Autodesk Fusion 360 part; units mm, degrees
(part 2 of 6)
sketch "mv_universal" plane through (-8.3287, 0, 77.2483) normal (0, 1, 0) x (1, 0, 0)
  line L0 (34.3787, 70.2483) -> (34.3787, 84.2483)
  line L1 (53.4287, 84.2483) -> (39.4287, 84.2483)
  line L2 (15.3287, 70.2483) -> (15.3287, 84.2483)
  line L3 (1.3287, 70.2483) -> (15.3287, 70.2483)
  line L4 (39.4287, 70.2483) -> (53.4287, 70.2483)
  line L5 (15.3287, 84.2483) -> (1.3287, 84.2483)
  line L6 (20.3787, 70.2483) -> (34.3787, 70.2483)
  line L7 (34.3787, 84.2483) -> (20.3787, 84.2483)
  line L8 (20.3787, 84.2483) -> (20.3787, 70.2483)
  line L9 (1.3287, 84.2483) -> (1.3287, 70.2483)
  line L10 (153.7287, 70.2483) -> (167.7287, 70.2483)
  line L11 (153.7287, 84.2483) -> (153.7287, 70.2483)
  line L12 (186.7787, 70.2483) -> (186.7787, 84.2483)
  line L13 (172.7787, 84.2483) -> (172.7787, 70.2483)
  line L14 (191.8287, 70.2483) -> (205.8287, 70.2483)
  line L15 (205.8287, 84.2483) -> (191.8287, 84.2483)
  line L16 (72.4787, 70.2483) -> (72.4787, 84.2483)
  line L17 (58.4787, 84.2483) -> (58.4787, 70.2483)
  line L18 (77.5287, 84.2483) -> (77.5287, 70.2483)
  line L19 (110.5787, 70.2483) -> (110.5787, 84.2483)
  line L20 (167.7287, 84.2483) -> (153.7287, 84.2483)
  line L21 (53.4287, 70.2483) -> (53.4287, 84.2483)
  line L22 (167.7287, 70.2483) -> (167.7287, 84.2483)
  line L23 (129.6287, 70.2483) -> (129.6287, 84.2483)
  line L24 (172.7787, 70.2483) -> (186.7787, 70.2483)
  line L25 (186.7787, 84.2483) -> (172.7787, 84.2483)
  line L26 (134.6787, 84.2483) -> (134.6787, 70.2483)
  line L27 (148.6787, 84.2483) -> (134.6787, 84.2483)
  line L28 (58.4787, 70.2483) -> (72.4787, 70.2483)
  line L29 (115.6287, 84.2483) -> (115.6287, 70.2483)
  line L30 (148.6787, 70.2483) -> (148.6787, 84.2483)
  line L31 (39.4287, 84.2483) -> (39.4287, 70.2483)
  line L32 (191.8287, 84.2483) -> (191.8287, 70.2483)
  line L33 (218.0224, 70.2483) -> (232.0224, 70.2483)
  line L34 (3.7099, 51.1983) -> (17.7099, 51.1983)
  line L35 (218.0224, 84.2483) -> (218.0224, 70.2483)
  line L36 (17.7099, 51.1983) -> (17.7099, 65.1983)
  line L37 (96.5787, 84.2483) -> (96.5787, 70.2483)
  line L38 (91.5287, 84.2483) -> (77.5287, 84.2483)
  line L39 (72.4787, 84.2483) -> (58.4787, 84.2483)
  line L40 (115.6287, 70.2483) -> (129.6287, 70.2483)
  line L41 (232.0224, 84.2483) -> (218.0224, 84.2483)
  line L42 (17.7099, 65.1983) -> (3.7099, 65.1983)
  line L43 (96.5787, 70.2483) -> (110.5787, 70.2483)
  line L44 (232.0224, 70.2483) -> (232.0224, 84.2483)
  line L45 (3.7099, 65.1983) -> (3.7099, 51.1983)
  line L46 (134.6787, 70.2483) -> (148.6787, 70.2483)
  line L47 (91.5287, 70.2483) -> (91.5287, 84.2483)
  line L48 (77.5287, 70.2483) -> (91.5287, 70.2483)
  line L49 (129.6287, 84.2483) -> (115.6287, 84.2483)
  line L50 (110.5787, 84.2483) -> (96.5787, 84.2483)
  line L51 (205.8287, 70.2483) -> (205.8287, 84.2483)
  line L52 (158.4912, 51.1983) -> (172.4912, 51.1983)
  line L53 (39.1412, 65.1983) -> (25.1412, 65.1983)
  line L54 (58.1912, 51.1983) -> (58.1912, 65.1983)
  line L55 (82.2912, 51.1983) -> (96.2912, 51.1983)
  line L56 (101.3412, 51.1983) -> (115.3412, 51.1983)
  line L57 (39.1412, 51.1983) -> (39.1412, 65.1983)
  line L58 (44.1912, 65.1983) -> (44.1912, 51.1983)
  line L59 (63.2412, 51.1983) -> (77.2412, 51.1983)
  line L60 (25.1412, 51.1983) -> (39.1412, 51.1983)
  line L61 (77.2412, 65.1983) -> (63.2412, 65.1983)
  line L62 (63.2412, 65.1983) -> (63.2412, 51.1983)
  line L63 (77.2412, 51.1983) -> (77.2412, 65.1983)
  line L64 (82.2912, 65.1983) -> (82.2912, 51.1983)
  line L65 (134.3912, 65.1983) -> (120.3912, 65.1983)
  line L66 (139.4412, 51.1983) -> (153.4412, 51.1983)
  line L67 (153.4412, 65.1983) -> (139.4412, 65.1983)
  line L68 (153.4412, 51.1983) -> (153.4412, 65.1983)
  line L69 (139.4412, 65.1983) -> (139.4412, 51.1983)
  line L70 (172.4912, 65.1983) -> (158.4912, 65.1983)
  line L71 (134.3912, 51.1983) -> (134.3912, 65.1983)
  line L72 (58.1912, 65.1983) -> (44.1912, 65.1983)
  line L73 (101.3412, 65.1983) -> (101.3412, 51.1983)
  line L74 (115.3412, 51.1983) -> (115.3412, 65.1983)
  line L75 (44.1912, 51.1983) -> (58.1912, 51.1983)
  line L76 (96.2912, 65.1983) -> (82.2912, 65.1983)
  line L77 (115.3412, 65.1983) -> (101.3412, 65.1983)
  line L78 (25.1412, 65.1983) -> (25.1412, 51.1983)
  line L79 (120.3912, 65.1983) -> (120.3912, 51.1983)
  line L80 (34.3787, 27.0983) -> (29.9037, 27.0983)
  line L81 (148.9662, 32.1483) -> (162.9662, 32.1483)
  line L82 (220.4037, 51.1983) -> (234.4037, 51.1983)
  line L83 (220.4037, 65.1983) -> (220.4037, 51.1983)
  line L84 (191.5412, 65.1983) -> (177.5412, 65.1983)
  line L85 (172.4912, 51.1983) -> (172.4912, 65.1983)
  line L86 (234.4037, 51.1983) -> (234.4037, 65.1983)
  line L87 (22.4724, 46.1483) -> (8.4724, 46.1483)
  line L88 (177.5412, 51.1983) -> (191.5412, 51.1983)
  line L89 (196.5912, 51.1983) -> (210.5912, 51.1983)
  line L90 (8.4724, 32.1483) -> (22.4724, 32.1483)
  line L91 (96.2912, 51.1983) -> (96.2912, 65.1983)
  line L92 (158.4912, 65.1983) -> (158.4912, 51.1983)
  line L93 (210.5912, 51.1983) -> (210.5912, 65.1983)
  line L94 (196.5912, 65.1983) -> (196.5912, 51.1983)
  line L95 (22.4724, 32.1483) -> (22.4724, 46.1483)
  line L96 (48.6662, 46.1483) -> (34.6662, 46.1483)
  line L97 (239.1662, 46.1483) -> (225.1662, 46.1483)
  line L98 (29.9037, 13.0983) -> (34.3787, 13.0983)
  line L99 (177.5412, 65.1983) -> (177.5412, 51.1983)
  line L100 (234.4037, 65.1983) -> (220.4037, 65.1983)
  line L101 (225.1662, 32.1483) -> (239.1662, 32.1483)
  line L102 (29.9037, 27.0983) -> (20.3787, 27.0983)
  line L103 (20.3787, 27.0983) -> (20.3787, 13.0983)
  line L104 (182.0162, 46.1483) -> (168.0162, 46.1483)
  line L105 (210.5912, 65.1983) -> (196.5912, 65.1983)
  line L106 (34.3787, 13.0983) -> (39.4287, 13.0983)
  line L107 (15.3287, 13.0983) -> (17.7099, 13.0983)
  line L108 (17.7099, 13.0983) -> (17.7099, 27.0983)
  line L109 (120.3912, 51.1983) -> (134.3912, 51.1983)
  line L110 (191.5412, 51.1983) -> (191.5412, 65.1983)
  line L111 (143.9162, 46.1483) -> (129.9162, 46.1483)
  line L112 (220.1162, 32.1483) -> (220.1162, 46.1483)
  line L113 (34.6662, 32.1483) -> (48.6662, 32.1483)
  line L114 (225.1662, 46.1483) -> (225.1662, 32.1483)
  line L115 (53.7162, 46.1483) -> (53.7162, 32.1483)
  line L116 (67.7162, 46.1483) -> (53.7162, 46.1483)
  line L117 (43.9037, 27.0983) -> (39.4287, 27.0983)
  line L118 (91.8162, 46.1483) -> (91.8162, 32.1483)
  line L119 (3.7099, 13.0983) -> (15.3287, 13.0983)
  line L120 (129.9162, 46.1483) -> (129.9162, 32.1483)
  line L121 (162.9662, 32.1483) -> (162.9662, 46.1483)
  line L122 (15.3287, 27.0983) -> (3.7099, 27.0983)
  line L123 (168.0162, 32.1483) -> (182.0162, 32.1483)
  line L124 (187.0662, 46.1483) -> (187.0662, 32.1483)
  line L125 (206.1162, 46.1483) -> (206.1162, 32.1483)
  line L126 (86.7662, 46.1483) -> (72.7662, 46.1483)
  line L127 (201.0662, 46.1483) -> (187.0662, 46.1483)
  line L128 (17.7099, 27.0983) -> (15.3287, 27.0983)
  line L129 (3.7099, 27.0983) -> (1.3287, 27.0983)
  line L130 (8.4724, 46.1483) -> (8.4724, 32.1483)
  line L131 (67.7162, 32.1483) -> (67.7162, 46.1483)
  line L132 (91.8162, 32.1483) -> (105.8162, 32.1483)
  line L133 (129.9162, 32.1483) -> (143.9162, 32.1483)
  line L134 (162.9662, 46.1483) -> (148.9662, 46.1483)
  line L135 (220.1162, 46.1483) -> (206.1162, 46.1483)
  line L136 (239.1662, 32.1483) -> (239.1662, 46.1483)
  line L137 (110.8662, 32.1483) -> (124.8662, 32.1483)
  line L138 (53.4287, 27.0983) -> (43.9037, 27.0983)
  line L139 (201.0662, 32.1483) -> (201.0662, 46.1483)
  line L140 (86.7662, 32.1483) -> (86.7662, 46.1483)
  line L141 (72.7662, 32.1483) -> (86.7662, 32.1483)
  line L142 (53.7162, 32.1483) -> (67.7162, 32.1483)
  line L143 (72.7662, 46.1483) -> (72.7662, 32.1483)
  line L144 (187.0662, 32.1483) -> (201.0662, 32.1483)
  line L145 (1.3287, 27.0983) -> (1.3287, 13.0983)
  line L146 (105.8162, 46.1483) -> (91.8162, 46.1483)
  line L147 (34.6662, 46.1483) -> (34.6662, 32.1483)
  line L148 (43.9037, 13.0983) -> (53.4287, 13.0983)
  line L149 (182.0162, 32.1483) -> (182.0162, 46.1483)
  line L150 (48.6662, 32.1483) -> (48.6662, 46.1483)
  line L151 (1.3287, 13.0983) -> (3.7099, 13.0983)
  line L152 (124.8662, 46.1483) -> (110.8662, 46.1483)
  line L153 (148.9662, 46.1483) -> (148.9662, 32.1483)
  line L154 (168.0162, 46.1483) -> (168.0162, 32.1483)
  line L155 (39.4287, 27.0983) -> (34.3787, 27.0983)
  line L156 (105.8162, 32.1483) -> (105.8162, 46.1483)
  line L157 (124.8662, 32.1483) -> (124.8662, 46.1483)
  line L158 (206.1162, 32.1483) -> (220.1162, 32.1483)
  line L159 (39.4287, 13.0983) -> (43.9037, 13.0983)
  line L160 (143.9162, 32.1483) -> (143.9162, 46.1483)
  line L161 (232.0224, 27.0983) -> (225.1662, 27.0983)
  line L162 (104.8729, 28.0983) -> (104.8729, 13.0983)
  line L163 (111.8729, 28.0983) -> (104.8729, 28.0983)
  line L164 (187.0662, 27.0983) -> (187.0662, 13.0983)
  line L165 (206.1162, 13.0983) -> (218.0224, 13.0983)
  line L166 (220.1162, 27.0983) -> (218.0224, 27.0983)
  line L167 (70.0974, 13.0983) -> (72.4787, 13.0983)
  line L168 (177.2537, 27.0983) -> (174.8724, 27.0983)
  line L169 (53.4287, 13.0983) -> (53.4287, 27.0983)
  line L170 (104.8729, 13.0983) -> (111.8729, 13.0983)
  line L171 (87.9969, 28.0983) -> (80.9969, 28.0983)
  line L172 (110.8662, 46.1483) -> (110.8662, 32.1483)
  line L173 (80.9969, 13.0983) -> (87.9969, 13.0983)
  line L174 (87.9969, 13.0983) -> (87.9969, 28.0983)
  line L175 (143.9162, 27.0983) -> (129.9162, 27.0983)
  line L176 (56.0974, 27.0983) -> (56.0974, 13.0983)
  line L177 (143.9162, 13.0983) -> (143.9162, 27.0983)
  line L178 (218.0224, 13.0983) -> (220.1162, 13.0983)
  line L179 (129.9162, 13.0983) -> (143.9162, 13.0983)
  line L180 (225.1662, 27.0983) -> (220.1162, 27.0983)
  line L181 (20.3787, 13.0983) -> (29.9037, 13.0983)
  line L182 (177.2537, 13.0983) -> (177.2537, 27.0983)
  line L183 (160.8724, 27.0983) -> (160.8724, 13.0983)
  line L184 (152.3542, 28.0983) -> (145.3542, 28.0983)
  line L185 (80.9969, 28.0983) -> (80.9969, 13.0983)
  line L186 (129.9162, 27.0983) -> (129.9162, 13.0983)
  line L187 (103.4349, 27.0983) -> (89.4349, 27.0983)
  line L188 (145.3542, 28.0983) -> (145.3542, 13.0983)
  line L189 (70.0974, 27.0983) -> (58.4787, 27.0983)
  line L190 (163.2537, 13.0983) -> (174.8724, 13.0983)
  line L191 (111.8729, 13.0983) -> (111.8729, 28.0983)
  line L192 (128.4782, 28.0983) -> (121.4782, 28.0983)
  line L193 (201.0662, 27.0983) -> (187.0662, 27.0983)
  line L194 (218.0224, 27.0983) -> (206.1162, 27.0983)
  line L195 (201.0662, 13.0983) -> (201.0662, 27.0983)
  line L196 (103.4349, 13.0983) -> (103.4349, 27.0983)
  line L197 (121.4782, 13.0983) -> (128.4782, 13.0983)
  line L198 (206.1162, 27.0983) -> (206.1162, 13.0983)
  line L199 (58.4787, 13.0983) -> (70.0974, 13.0983)
  line L200 (239.1662, 27.0983) -> (232.0224, 27.0983)
  line L201 (187.0662, 13.0983) -> (201.0662, 13.0983)
  line L202 (145.3542, 13.0983) -> (152.3542, 13.0983)
  line L203 (72.4787, 13.0983) -> (72.4787, 27.0983)
  line L204 (152.3542, 13.0983) -> (152.3542, 28.0983)
  line L205 (174.8724, 13.0983) -> (177.2537, 13.0983)
  line L206 (58.4787, 27.0983) -> (56.0974, 27.0983)
  line L207 (225.1662, 13.0983) -> (232.0224, 13.0983)
  line L208 (56.0974, 13.0983) -> (58.4787, 13.0983)
  line L209 (89.4349, 27.0983) -> (89.4349, 13.0983)
  line L210 (72.4787, 27.0983) -> (70.0974, 27.0983)
  line L211 (232.0224, 13.0983) -> (239.1662, 13.0983)
  line L212 (121.4782, 28.0983) -> (121.4782, 13.0983)
  line L213 (239.1662, 13.0983) -> (239.1662, 27.0983)
  line L214 (89.4349, 13.0983) -> (103.4349, 13.0983)
  line L215 (163.2537, 27.0983) -> (160.8724, 27.0983)
  line L216 (128.4782, 13.0983) -> (128.4782, 28.0983)
  line L217 (174.8724, 27.0983) -> (163.2537, 27.0983)
  line L218 (220.1162, 13.0983) -> (225.1662, 13.0983)
  line L219 (160.8724, 13.0983) -> (163.2537, 13.0983)
  point P0 (8.3287, 77.2483)
sketch "monorail_steam" plane through (-2.7257, 0, 77.6837) normal (0, 1, 0) x (1, 0, 0)
  line L0 (228.8007, 51.6337) -> (228.8007, 65.6337)
  line L1 (43.0632, 32.5837) -> (43.0632, 46.5837)
  line L2 (188.3195, 27.5337) -> (176.7007, 27.5337)
  line L3 (29.0632, 46.5837) -> (29.0632, 32.5837)
  line L4 (138.3132, 32.5837) -> (138.3132, 46.5837)
  line L5 (157.3632, 32.5837) -> (157.3632, 46.5837)
  line L6 (119.2632, 46.5837) -> (105.2632, 46.5837)
  line L7 (209.7507, 27.5337) -> (195.7507, 27.5337)
  line L8 (190.7007, 27.5337) -> (188.3195, 27.5337)
  line L9 (217.182, 27.5337) -> (217.182, 13.5337)
  line L10 (195.7507, 13.5337) -> (209.7507, 13.5337)
  line L11 (190.7007, 13.5337) -> (190.7007, 27.5337)
  line L12 (118.2882, 28.5337) -> (118.2882, 27.5337)
  line L13 (174.3195, 13.5337) -> (176.7007, 13.5337)
  line L14 (231.182, 13.5337) -> (231.182, 27.5337)
  line L15 (217.182, 13.5337) -> (231.182, 13.5337)
  line L16 (174.3195, 27.5337) -> (174.3195, 13.5337)
  line L17 (231.182, 27.5337) -> (217.182, 27.5337)
  line L18 (188.3195, 13.5337) -> (190.7007, 13.5337)
  line L19 (125.2882, 13.5337) -> (125.2882, 28.5337)
  line L20 (195.7507, 27.5337) -> (195.7507, 13.5337)
  line L21 (176.7007, 13.5337) -> (188.3195, 13.5337)
  line L22 (209.7507, 13.5337) -> (209.7507, 27.5337)
  line L23 (176.7007, 27.5337) -> (174.3195, 27.5337)
  line L24 (105.2632, 32.5837) -> (119.2632, 32.5837)
  line L25 (2.8695, 32.5837) -> (16.8695, 32.5837)
  line L26 (162.4132, 32.5837) -> (176.4132, 32.5837)
  line L27 (204.9882, 65.6337) -> (190.9882, 65.6337)
  line L28 (176.4132, 46.5837) -> (162.4132, 46.5837)
  line L29 (62.1132, 46.5837) -> (48.1132, 46.5837)
  line L30 (124.3132, 46.5837) -> (124.3132, 32.5837)
  line L31 (62.1132, 32.5837) -> (62.1132, 46.5837)
  line L32 (195.4632, 46.5837) -> (181.4632, 46.5837)
  line L33 (138.3132, 46.5837) -> (124.3132, 46.5837)
  line L34 (48.1132, 46.5837) -> (48.1132, 32.5837)
  line L35 (105.2632, 46.5837) -> (105.2632, 32.5837)
  line L36 (166.8882, 51.6337) -> (166.8882, 65.6337)
  line L37 (67.1632, 32.5837) -> (81.1632, 32.5837)
  line L38 (171.9382, 51.6337) -> (185.9382, 51.6337)
  line L39 (100.2132, 32.5837) -> (100.2132, 46.5837)
  line L40 (219.5632, 32.5837) -> (233.5632, 32.5837)
  line L41 (176.4132, 32.5837) -> (176.4132, 46.5837)
  line L42 (181.4632, 32.5837) -> (195.4632, 32.5837)
  line L43 (100.2132, 46.5837) -> (86.2132, 46.5837)
  line L44 (200.5132, 32.5837) -> (214.5132, 32.5837)
  line L45 (162.4132, 46.5837) -> (162.4132, 32.5837)
  line L46 (190.9882, 65.6337) -> (190.9882, 51.6337)
  line L47 (29.0632, 32.5837) -> (43.0632, 32.5837)
  line L48 (86.2132, 46.5837) -> (86.2132, 32.5837)
  line L49 (43.0632, 46.5837) -> (29.0632, 46.5837)
  line L50 (185.9382, 51.6337) -> (185.9382, 65.6337)
  line L51 (171.9382, 65.6337) -> (171.9382, 51.6337)
  line L52 (16.8695, 32.5837) -> (16.8695, 46.5837)
  line L53 (124.3132, 32.5837) -> (138.3132, 32.5837)
  line L54 (185.9382, 65.6337) -> (171.9382, 65.6337)
  line L55 (81.1632, 32.5837) -> (81.1632, 46.5837)
  line L56 (228.8007, 65.6337) -> (214.8007, 65.6337)
  line L57 (166.8882, 65.6337) -> (152.8882, 65.6337)
  line L58 (57.6382, 65.6337) -> (57.6382, 51.6337)
  line L59 (133.8382, 65.6337) -> (133.8382, 51.6337)
  line L60 (152.8882, 51.6337) -> (166.8882, 51.6337)
  line L61 (133.8382, 51.6337) -> (147.8382, 51.6337)
  line L62 (90.6882, 65.6337) -> (76.6882, 65.6337)
  line L63 (76.6882, 65.6337) -> (76.6882, 51.6337)
  line L64 (95.7382, 51.6337) -> (109.7382, 51.6337)
  line L65 (109.7382, 65.6337) -> (95.7382, 65.6337)
  line L66 (95.7382, 65.6337) -> (95.7382, 51.6337)
  line L67 (128.7882, 51.6337) -> (128.7882, 65.6337)
  line L68 (147.8382, 51.6337) -> (147.8382, 65.6337)
  line L69 (214.8007, 65.6337) -> (214.8007, 51.6337)
  line L70 (114.7882, 65.6337) -> (114.7882, 51.6337)
  line L71 (109.7382, 51.6337) -> (109.7382, 65.6337)
  line L72 (128.7882, 65.6337) -> (114.7882, 65.6337)
  line L73 (90.6882, 51.6337) -> (90.6882, 65.6337)
  line L74 (114.7882, 51.6337) -> (128.7882, 51.6337)
  line L75 (147.8382, 65.6337) -> (133.8382, 65.6337)
  line L76 (76.6882, 51.6337) -> (90.6882, 51.6337)
  line L77 (143.3632, 46.5837) -> (143.3632, 32.5837)
  line L78 (195.4632, 32.5837) -> (195.4632, 46.5837)
  line L79 (143.3632, 32.5837) -> (157.3632, 32.5837)
  line L80 (181.4632, 46.5837) -> (181.4632, 32.5837)
  line L81 (16.8695, 46.5837) -> (2.8695, 46.5837)
  line L82 (152.8882, 65.6337) -> (152.8882, 51.6337)
  line L83 (214.8007, 51.6337) -> (228.8007, 51.6337)
  line L84 (214.5132, 46.5837) -> (200.5132, 46.5837)
  line L85 (157.3632, 46.5837) -> (143.3632, 46.5837)
  line L86 (67.1632, 46.5837) -> (67.1632, 32.5837)
  line L87 (190.9882, 51.6337) -> (204.9882, 51.6337)
  line L88 (214.5132, 32.5837) -> (214.5132, 46.5837)
  line L89 (86.2132, 32.5837) -> (100.2132, 32.5837)
  line L90 (81.1632, 46.5837) -> (67.1632, 46.5837)
  line L91 (119.2632, 32.5837) -> (119.2632, 46.5837)
  line L92 (200.5132, 46.5837) -> (200.5132, 32.5837)
  line L93 (233.5632, 46.5837) -> (219.5632, 46.5837)
  line L94 (219.5632, 46.5837) -> (219.5632, 32.5837)
  line L95 (204.9882, 51.6337) -> (204.9882, 65.6337)
  line L96 (2.8695, 46.5837) -> (2.8695, 32.5837)
  line L97 (233.5632, 32.5837) -> (233.5632, 46.5837)
  line L98 (48.1132, 32.5837) -> (62.1132, 32.5837)
  line L99 (110.0257, 70.6837) -> (124.0257, 70.6837)
  line L100 (181.1757, 84.6837) -> (167.1757, 84.6837)
  line L101 (85.9257, 84.6837) -> (71.9257, 84.6837)
  line L102 (124.0257, 70.6837) -> (124.0257, 84.6837)
  line L103 (129.0757, 70.6837) -> (143.0757, 70.6837)
  line L104 (162.1257, 70.6837) -> (162.1257, 84.6837)
  line L105 (52.8757, 70.6837) -> (66.8757, 70.6837)
  line L106 (28.7757, 84.6837) -> (14.7757, 84.6837)
  line L107 (162.1257, 84.6837) -> (148.1257, 84.6837)
  line L108 (-4.2743, 70.6837) -> (9.7257, 70.6837)
  line L109 (28.7757, 70.6837) -> (28.7757, 84.6837)
  line L110 (148.1257, 84.6837) -> (148.1257, 70.6837)
  line L111 (167.1757, 84.6837) -> (167.1757, 70.6837)
  line L112 (71.9257, 70.6837) -> (85.9257, 70.6837)
  line L113 (47.8257, 70.6837) -> (47.8257, 84.6837)
  line L114 (85.9257, 70.6837) -> (85.9257, 84.6837)
  line L115 (90.9757, 70.6837) -> (104.9757, 70.6837)
  line L116 (14.7757, 84.6837) -> (14.7757, 70.6837)
  line L117 (71.9257, 84.6837) -> (71.9257, 70.6837)
  line L118 (52.8757, 84.6837) -> (52.8757, 70.6837)
  line L119 (104.9757, 84.6837) -> (90.9757, 84.6837)
  line L120 (110.0257, 84.6837) -> (110.0257, 70.6837)
  line L121 (90.9757, 84.6837) -> (90.9757, 70.6837)
  line L122 (104.9757, 70.6837) -> (104.9757, 84.6837)
  line L123 (47.8257, 84.6837) -> (33.8257, 84.6837)
  line L124 (212.4195, 70.6837) -> (226.4195, 70.6837)
  line L125 (226.4195, 84.6837) -> (212.4195, 84.6837)
  line L126 (226.4195, 70.6837) -> (226.4195, 84.6837)
  line L127 (200.2257, 70.6837) -> (200.2257, 84.6837)
  line L128 (186.2257, 84.6837) -> (186.2257, 70.6837)
  line L129 (-1.893, 51.6337) -> (12.107, 51.6337)
  line L130 (12.107, 51.6337) -> (12.107, 65.6337)
  line L131 (33.5382, 65.6337) -> (19.5382, 65.6337)
  line L132 (19.5382, 65.6337) -> (19.5382, 51.6337)
  line L133 (38.5882, 51.6337) -> (52.5882, 51.6337)
  line L134 (212.4195, 84.6837) -> (212.4195, 70.6837)
  line L135 (-1.893, 65.6337) -> (-1.893, 51.6337)
  line L136 (12.107, 65.6337) -> (-1.893, 65.6337)
  line L137 (19.5382, 51.6337) -> (33.5382, 51.6337)
  line L138 (33.5382, 51.6337) -> (33.5382, 65.6337)
  line L139 (52.5882, 65.6337) -> (38.5882, 65.6337)
  line L140 (38.5882, 65.6337) -> (38.5882, 51.6337)
  line L141 (52.5882, 51.6337) -> (52.5882, 65.6337)
  line L142 (71.6382, 65.6337) -> (57.6382, 65.6337)
  line L143 (57.6382, 51.6337) -> (71.6382, 51.6337)
  line L144 (71.6382, 51.6337) -> (71.6382, 65.6337)
  line L145 (9.7257, 70.6837) -> (9.7257, 84.6837)
  line L146 (33.8257, 84.6837) -> (33.8257, 70.6837)
  line L147 (14.7757, 70.6837) -> (28.7757, 70.6837)
  line L148 (66.8757, 70.6837) -> (66.8757, 84.6837)
  line L149 (61.1445, 13.5337) -> (68.1382, 13.5337)
  line L150 (118.2882, 13.5337) -> (121.6445, 13.5337)
  line L151 (33.5382, 13.5337) -> (33.5382, 27.5337)
  line L152 (76.6882, 13.5337) -> (77.6315, 13.5337)
  line L153 (19.5382, 27.5337) -> (17.157, 27.5337)
  line L154 (168.1445, 13.5337) -> (168.1445, 28.5337)
  line L155 (121.6445, 13.5337) -> (125.2882, 13.5337)
  line L156 (38.5882, 27.5337) -> (38.5882, 13.5337)
  line L157 (106.2382, 28.5337) -> (101.5075, 28.5337)
  line L158 (61.1382, 28.5337) -> (61.1382, 13.5337)
  line L159 (156.3882, 13.5337) -> (161.1445, 13.5337)
  line L160 (133.8382, 27.5337) -> (133.8382, 13.5337)
  line L161 (33.5382, 27.5337) -> (31.157, 27.5337)
  line L162 (61.1445, 28.5337) -> (61.1382, 28.5337)
  line L163 (156.3882, 28.5337) -> (156.3882, 13.5337)
  line L164 (125.2882, 28.5337) -> (118.2882, 28.5337)
  line L165 (161.1445, 28.5337) -> (156.3882, 28.5337)
  line L166 (61.1382, 13.5337) -> (61.1445, 13.5337)
  line L167 (107.6445, 13.5337) -> (118.2882, 13.5337)
  line L168 (147.8382, 27.5337) -> (133.8382, 27.5337)
  line L169 (-4.2743, 27.5337) -> (-4.2743, 13.5337)
  line L170 (94.5075, 28.5337) -> (94.5075, 13.5337)
  line L171 (54.9695, 13.5337) -> (54.9695, 27.5337)
  line L172 (68.1445, 28.5337) -> (68.1382, 28.5337)
  line L173 (77.6315, 28.5337) -> (70.6315, 28.5337)
  line L174 (99.2382, 28.5337) -> (94.5075, 28.5337)
  line L175 (17.157, 27.5337) -> (17.157, 13.5337)
  line L176 (40.9695, 27.5337) -> (38.5882, 27.5337)
  line L177 (40.9695, 13.5337) -> (52.5882, 13.5337)
  line L178 (118.2882, 27.5337) -> (107.6445, 27.5337)
  line L179 (168.1445, 28.5337) -> (163.3882, 28.5337)
  line L180 (31.157, 13.5337) -> (33.5382, 13.5337)
  line L181 (101.5075, 13.5337) -> (106.2382, 13.5337)
  line L182 (107.6445, 27.5337) -> (107.6445, 13.5337)
  line L183 (68.1445, 13.5337) -> (68.1445, 28.5337)
  line L184 (70.6315, 28.5337) -> (70.6315, 13.5337)
  line L185 (90.6882, 13.5337) -> (93.0695, 13.5337)
  line L186 (77.6315, 27.5337) -> (77.6315, 28.5337)
  line L187 (68.1382, 13.5337) -> (68.1445, 13.5337)
  line L188 (133.8382, 13.5337) -> (147.8382, 13.5337)
  line L189 (147.8382, 13.5337) -> (147.8382, 27.5337)
  line L190 (9.7257, 13.5337) -> (12.107, 13.5337)
  line L191 (-4.2743, 13.5337) -> (-1.893, 13.5337)
  line L192 (77.6315, 13.5337) -> (79.0695, 13.5337)
  line L193 (-1.893, 13.5337) -> (9.7257, 13.5337)
  line L194 (54.9695, 27.5337) -> (52.5882, 27.5337)
  line L195 (94.5075, 13.5337) -> (99.2382, 13.5337)
  line L196 (12.107, 13.5337) -> (12.107, 27.5337)
  line L197 (93.0695, 27.5337) -> (90.6882, 27.5337)
  line L198 (93.0695, 13.5337) -> (93.0695, 27.5337)
  line L199 (70.6315, 13.5337) -> (76.6882, 13.5337)
  line L200 (52.5882, 27.5337) -> (40.9695, 27.5337)
  line L201 (101.5075, 28.5337) -> (99.2382, 28.5337)
  line L202 (68.1382, 28.5337) -> (61.1445, 28.5337)
  line L203 (19.5382, 13.5337) -> (31.157, 13.5337)
  line L204 (79.0695, 13.5337) -> (90.6882, 13.5337)
  line L205 (163.3882, 13.5337) -> (168.1445, 13.5337)
  line L206 (9.7257, 27.5337) -> (-1.893, 27.5337)
  line L207 (90.6882, 27.5337) -> (79.0695, 27.5337)
  line L208 (31.157, 27.5337) -> (19.5382, 27.5337)
  line L209 (106.2382, 13.5337) -> (106.2382, 28.5337)
  line L210 (17.157, 13.5337) -> (19.5382, 13.5337)
  line L211 (12.107, 27.5337) -> (9.7257, 27.5337)
  line L212 (79.0695, 27.5337) -> (77.6315, 27.5337)
  line L213 (-1.893, 27.5337) -> (-4.2743, 27.5337)
  line L214 (38.5882, 13.5337) -> (40.9695, 13.5337)
  line L215 (52.5882, 13.5337) -> (54.9695, 13.5337)
  line L216 (161.1445, 13.5337) -> (163.3882, 13.5337)
  line L217 (99.2382, 13.5337) -> (101.5075, 13.5337)
  line L218 (163.3882, 28.5337) -> (161.1445, 28.5337)
  line L219 (129.0757, 84.6837) -> (129.0757, 70.6837)
  line L220 (143.0757, 84.6837) -> (129.0757, 84.6837)
  line L221 (181.1757, 70.6837) -> (181.1757, 84.6837)
  line L222 (124.0257, 84.6837) -> (110.0257, 84.6837)
  line L223 (167.1757, 70.6837) -> (181.1757, 70.6837)
  line L224 (186.2257, 70.6837) -> (200.2257, 70.6837)
  line L225 (200.2257, 84.6837) -> (186.2257, 84.6837)
  line L226 (143.0757, 70.6837) -> (143.0757, 84.6837)
  line L227 (9.7257, 84.6837) -> (-4.2743, 84.6837)
  line L228 (66.8757, 84.6837) -> (52.8757, 84.6837)
  line L229 (148.1257, 70.6837) -> (162.1257, 70.6837)
  line L230 (33.8257, 70.6837) -> (47.8257, 70.6837)
  line L231 (-4.2743, 84.6837) -> (-4.2743, 70.6837)
  point P0 (2.7257, 77.6837)
sketch "monorail_universal" plane through (-6.4028, 0, 77.4536) normal (0, 1, 0) x (1, 0, 0)
  line L0 (113.4153, 65.4036) -> (99.4153, 65.4036)
  line L1 (20.5466, 32.3536) -> (20.5466, 46.3536)
  line L2 (194.6653, 65.4036) -> (194.6653, 51.4036)
  line L3 (218.4778, 65.4036) -> (218.4778, 51.4036)
  line L4 (94.3653, 51.4036) -> (94.3653, 65.4036)
  line L5 (32.7403, 46.3536) -> (32.7403, 32.3536)
  line L6 (27.9778, 27.3036) -> (23.2153, 27.3036)
  line L7 (61.3153, 65.4036) -> (61.3153, 51.4036)
  line L8 (175.6153, 65.4036) -> (175.6153, 51.4036)
  line L9 (103.8903, 32.3536) -> (103.8903, 46.3536)
  line L10 (189.6153, 51.4036) -> (189.6153, 65.4036)
  line L11 (137.5153, 65.4036) -> (137.5153, 51.4036)
  line L12 (54.1716, 27.3036) -> (51.5028, 27.3036)
  line L13 (199.1403, 46.3536) -> (185.1403, 46.3536)
  line L14 (204.1903, 46.3536) -> (204.1903, 32.3536)
  line L15 (185.1403, 32.3536) -> (199.1403, 32.3536)
  line L16 (64.8153, 13.3036) -> (64.8216, 13.3036)
  line L17 (223.2403, 46.3536) -> (223.2403, 32.3536)
  line L18 (27.9778, 13.3036) -> (32.4528, 13.3036)
  line L19 (237.2403, 46.3536) -> (223.2403, 46.3536)
  line L20 (199.1403, 32.3536) -> (199.1403, 46.3536)
  line L21 (68.1716, 13.3036) -> (69.5841, 13.3036)
  line L22 (56.2653, 13.3036) -> (56.5528, 13.3036)
  line L23 (180.0903, 32.3536) -> (180.0903, 46.3536)
  line L24 (34.8341, 13.3036) -> (37.2153, 13.3036)
  line L25 (-0.5972, 13.3036) -> (1.7841, 13.3036)
  line L26 (185.1403, 46.3536) -> (185.1403, 32.3536)
  line L27 (44.6466, 27.3036) -> (42.2653, 27.3036)
  line L28 (42.2653, 27.3036) -> (41.9778, 27.3036)
  line L29 (23.2153, 27.3036) -> (20.8341, 27.3036)
  line L30 (34.8341, 27.3036) -> (32.4528, 27.3036)
  line L31 (161.0403, 46.3536) -> (147.0403, 46.3536)
  line L32 (37.5028, 27.3036) -> (37.2153, 27.3036)
  line L33 (42.2653, 13.3036) -> (44.6466, 13.3036)
  line L34 (15.7841, 13.3036) -> (15.7841, 27.3036)
  line L35 (37.5028, 13.3036) -> (41.9778, 13.3036)
  line L36 (204.1903, 32.3536) -> (218.1903, 32.3536)
  line L37 (15.7841, 27.3036) -> (13.4028, 27.3036)
  line L38 (180.0903, 46.3536) -> (166.0903, 46.3536)
  line L39 (161.0403, 32.3536) -> (161.0403, 46.3536)
  line L40 (56.5528, 13.3036) -> (58.6466, 13.3036)
  line L41 (147.0403, 46.3536) -> (147.0403, 32.3536)
  line L42 (13.4028, 27.3036) -> (1.7841, 27.3036)
  line L43 (-0.5972, 27.3036) -> (-0.5972, 13.3036)
  line L44 (37.2153, 13.3036) -> (37.5028, 13.3036)
  line L45 (23.2153, 13.3036) -> (27.9778, 13.3036)
  line L46 (1.7841, 13.3036) -> (13.4028, 13.3036)
  line L47 (41.9778, 27.3036) -> (37.5028, 27.3036)
  line L48 (37.2153, 27.3036) -> (34.8341, 27.3036)
  line L49 (32.4528, 13.3036) -> (34.8341, 13.3036)
  line L50 (32.4528, 27.3036) -> (27.9778, 27.3036)
  line L51 (20.8341, 27.3036) -> (18.4528, 27.3036)
  line L52 (223.2403, 32.3536) -> (237.2403, 32.3536)
  line L53 (166.0903, 32.3536) -> (180.0903, 32.3536)
  line L54 (166.0903, 46.3536) -> (166.0903, 32.3536)
  line L55 (56.2653, 27.3036) -> (54.1716, 27.3036)
  line L56 (44.6466, 13.3036) -> (51.5028, 13.3036)
  line L57 (237.2403, 32.3536) -> (237.2403, 46.3536)
  line L58 (58.6466, 27.3036) -> (56.5528, 27.3036)
  line L59 (54.1716, 13.3036) -> (56.2653, 13.3036)
  line L60 (41.9778, 13.3036) -> (42.2653, 13.3036)
  line L61 (51.5028, 27.3036) -> (44.6466, 27.3036)
  line L62 (58.6466, 13.3036) -> (64.8153, 13.3036)
  line L63 (18.4528, 13.3036) -> (20.8341, 13.3036)
  line L64 (218.1903, 46.3536) -> (204.1903, 46.3536)
  line L65 (171.8216, 28.3036) -> (169.5841, 28.3036)
  line L66 (111.3216, 13.3036) -> (116.0841, 13.3036)
  line L67 (56.5528, 27.3036) -> (56.2653, 27.3036)
  line L68 (116.0841, 27.3036) -> (111.3216, 27.3036)
  line L69 (20.8341, 13.3036) -> (23.2153, 13.3036)
  line L70 (51.5028, 13.3036) -> (54.1716, 13.3036)
  line L71 (218.1903, 32.3536) -> (218.1903, 46.3536)
  line L72 (176.5841, 28.3036) -> (171.8216, 28.3036)
  line L73 (176.5841, 27.3036) -> (176.5841, 28.3036)
  line L74 (98.1846, 13.3036) -> (101.5091, 13.3036)
  line L75 (1.7841, 27.3036) -> (-0.5972, 27.3036)
  line L76 (64.8153, 28.3036) -> (64.8153, 27.3036)
  line L77 (74.3086, 13.3036) -> (76.5841, 13.3036)
  line L78 (71.8153, 13.3036) -> (71.8216, 13.3036)
  line L79 (121.9653, 13.3036) -> (125.3216, 13.3036)
  line L80 (18.4528, 27.3036) -> (18.4528, 13.3036)
  line L81 (172.9466, 13.3036) -> (173.2341, 13.3036)
  line L82 (79.0711, 13.3036) -> (80.3653, 13.3036)
  line L83 (79.0711, 28.3036) -> (76.5841, 28.3036)
  line L84 (126.5523, 13.3036) -> (127.9903, 13.3036)
  line L85 (81.3086, 28.3036) -> (79.0711, 28.3036)
  line L86 (164.8216, 13.3036) -> (167.0653, 13.3036)
  line L87 (82.7466, 13.3036) -> (86.0711, 13.3036)
  line L88 (71.8153, 28.3036) -> (69.5841, 28.3036)
  line L89 (69.5841, 28.3036) -> (64.8216, 28.3036)
  line L90 (109.9153, 28.3036) -> (105.1846, 28.3036)
  line L91 (102.9153, 13.3036) -> (102.9471, 13.3036)
  line L92 (105.1846, 13.3036) -> (109.9153, 13.3036)
  line L93 (76.5841, 28.3036) -> (74.3086, 28.3036)
  line L94 (87.5091, 13.3036) -> (94.3653, 13.3036)
  line L95 (64.8216, 28.3036) -> (64.8153, 28.3036)
  line L96 (169.5841, 28.3036) -> (167.0653, 28.3036)
  line L97 (101.5091, 13.3036) -> (102.9153, 13.3036)
  line L98 (98.1846, 28.3036) -> (98.1846, 27.3036)
  line L99 (116.0841, 13.3036) -> (119.5523, 13.3036)
  line L100 (94.3653, 27.3036) -> (87.5091, 27.3036)
  line L101 (105.1846, 28.3036) -> (102.9471, 28.3036)
  line L102 (102.9471, 13.3036) -> (105.1846, 13.3036)
  line L103 (64.8153, 27.3036) -> (58.6466, 27.3036)
  line L104 (13.4028, 13.3036) -> (15.7841, 13.3036)
  line L105 (69.5841, 13.3036) -> (70.5528, 13.3036)
  line L106 (64.8216, 13.3036) -> (68.1716, 13.3036)
  line L107 (94.3653, 13.3036) -> (96.7466, 13.3036)
  line L108 (71.8216, 28.3036) -> (71.8153, 28.3036)
  line L109 (86.0711, 13.3036) -> (87.5091, 13.3036)
  line L110 (76.5841, 13.3036) -> (79.0711, 13.3036)
  line L111 (119.5523, 27.3036) -> (116.0841, 27.3036)
  line L112 (173.2341, 13.3036) -> (175.3278, 13.3036)
  line L113 (87.5091, 27.3036) -> (86.0711, 27.3036)
  line L114 (102.9153, 28.3036) -> (98.1846, 28.3036)
  line L115 (111.3216, 27.3036) -> (111.3216, 13.3036)
  line L116 (128.9336, 13.3036) -> (128.9653, 13.3036)
  line L117 (80.3653, 13.3036) -> (81.3086, 13.3036)
  line L118 (128.9653, 27.3036) -> (128.9653, 28.3036)
  line L119 (180.3778, 13.3036) -> (185.1403, 13.3036)
  line L120 (175.3278, 13.3036) -> (176.5841, 13.3036)
  line L121 (145.8096, 28.3036) -> (143.4283, 28.3036)
  line L122 (213.4278, 13.3036) -> (216.0966, 13.3036)
  line L123 (144.3716, 13.3036) -> (145.8096, 13.3036)
  line L124 (185.1403, 13.3036) -> (187.2341, 13.3036)
  line L125 (161.3278, 13.3036) -> (163.7091, 13.3036)
  line L126 (130.0841, 27.3036) -> (128.9653, 27.3036)
  line L127 (167.0653, 13.3036) -> (169.5841, 13.3036)
  line L128 (98.1846, 27.3036) -> (96.7466, 27.3036)
  line L129 (177.7091, 27.3036) -> (176.5841, 27.3036)
  line L130 (177.9966, 27.3036) -> (177.7091, 27.3036)
  line L131 (70.5528, 13.3036) -> (71.8153, 13.3036)
  line L132 (164.8216, 28.3036) -> (160.0653, 28.3036)
  line L133 (187.2341, 13.3036) -> (189.9028, 13.3036)
  line L134 (171.8216, 13.3036) -> (172.9466, 13.3036)
  line L135 (191.9966, 27.3036) -> (189.9028, 27.3036)
  line L136 (191.9966, 13.3036) -> (194.3778, 13.3036)
  line L137 (151.5153, 13.3036) -> (152.8096, 13.3036)
  line L138 (143.4283, 28.3036) -> (143.4283, 27.3036)
  line L139 (152.8096, 28.3036) -> (150.4283, 28.3036)
  line L140 (96.7466, 27.3036) -> (94.3653, 27.3036)
  line L141 (71.8216, 13.3036) -> (74.3086, 13.3036)
  line L142 (119.5523, 13.3036) -> (121.9336, 13.3036)
  line L143 (160.0653, 28.3036) -> (160.0653, 27.3036)
  line L144 (96.7466, 13.3036) -> (98.1846, 13.3036)
  line L145 (109.9153, 13.3036) -> (109.9471, 13.3036)
  line L146 (167.0653, 28.3036) -> (164.8216, 28.3036)
  line L147 (127.9903, 13.3036) -> (128.9336, 13.3036)
  line L148 (81.3086, 13.3036) -> (82.7466, 13.3036)
  line L149 (216.0966, 13.3036) -> (218.1903, 13.3036)
  line L150 (152.8096, 13.3036) -> (152.8096, 28.3036)
  line L151 (177.9966, 13.3036) -> (180.3778, 13.3036)
  line L152 (102.9471, 28.3036) -> (102.9153, 28.3036)
  line L153 (169.5841, 13.3036) -> (171.8216, 13.3036)
  line L154 (109.9471, 28.3036) -> (109.9153, 28.3036)
  line L155 (125.3216, 13.3036) -> (126.5523, 13.3036)
  line L156 (121.9336, 13.3036) -> (121.9653, 13.3036)
  line L157 (74.3086, 28.3036) -> (71.8216, 28.3036)
  line L158 (128.9653, 13.3036) -> (130.0841, 13.3036)
  line L159 (128.9653, 28.3036) -> (128.9336, 28.3036)
  line L160 (199.1403, 27.3036) -> (194.3778, 27.3036)
  line L161 (163.7091, 13.3036) -> (164.8216, 13.3036)
  line L162 (121.9653, 28.3036) -> (121.9336, 28.3036)
  line L163 (160.0653, 13.3036) -> (161.3278, 13.3036)
  line L164 (177.7091, 13.3036) -> (177.9966, 13.3036)
  line L165 (189.9028, 13.3036) -> (191.9966, 13.3036)
  line L166 (121.9336, 28.3036) -> (119.5523, 28.3036)
  line L167 (194.3778, 13.3036) -> (199.1403, 13.3036)
  line L168 (150.4283, 13.3036) -> (151.5153, 13.3036)
  line L169 (141.9903, 13.3036) -> (143.4283, 13.3036)
  line L170 (137.5153, 13.3036) -> (141.9903, 13.3036)
  line L171 (187.2341, 27.3036) -> (185.1403, 27.3036)
  line L172 (203.9028, 13.3036) -> (204.1903, 13.3036)
  line L173 (158.9466, 13.3036) -> (160.0653, 13.3036)
  line L174 (185.1403, 27.3036) -> (180.3778, 27.3036)
  line L175 (130.3716, 13.3036) -> (137.5153, 13.3036)
  line L176 (180.3778, 27.3036) -> (177.9966, 27.3036)
  line L177 (130.3716, 27.3036) -> (130.0841, 27.3036)
  line L178 (143.4283, 27.3036) -> (141.9903, 27.3036)
  line L179 (145.8096, 13.3036) -> (150.4283, 13.3036)
  line L180 (143.4283, 13.3036) -> (144.3716, 13.3036)
  line L181 (128.9336, 28.3036) -> (126.5523, 28.3036)
  line L182 (199.4278, 13.3036) -> (203.9028, 13.3036)
  line L183 (126.5523, 28.3036) -> (121.9653, 28.3036)
  line L184 (119.5523, 28.3036) -> (119.5523, 27.3036)
  line L185 (150.4283, 28.3036) -> (145.8096, 28.3036)
  line L186 (189.9028, 27.3036) -> (187.2341, 27.3036)
  line L187 (158.9466, 27.3036) -> (158.9466, 13.3036)
  line L188 (203.9028, 27.3036) -> (199.4278, 27.3036)
  line L189 (176.5841, 13.3036) -> (177.7091, 13.3036)
  line L190 (141.9903, 27.3036) -> (137.5153, 27.3036)
  line L191 (213.4278, 27.3036) -> (204.1903, 27.3036)
  line L192 (204.1903, 27.3036) -> (203.9028, 27.3036)
  line L193 (130.0841, 13.3036) -> (130.3716, 13.3036)
  line L194 (194.3778, 27.3036) -> (191.9966, 27.3036)
  line L195 (204.1903, 13.3036) -> (213.4278, 13.3036)
  line L196 (199.4278, 27.3036) -> (199.1403, 27.3036)
  line L197 (86.0711, 27.3036) -> (86.0711, 28.3036)
  line L198 (86.0711, 28.3036) -> (81.3086, 28.3036)
  line L199 (160.0653, 27.3036) -> (158.9466, 27.3036)
  line L200 (109.9471, 13.3036) -> (109.9471, 28.3036)
  line L201 (199.1403, 13.3036) -> (199.4278, 13.3036)
  line L202 (234.8591, 27.3036) -> (230.0966, 27.3036)
  line L203 (137.5153, 27.3036) -> (130.3716, 27.3036)
  line L204 (220.8591, 13.3036) -> (223.2403, 13.3036)
  line L205 (220.8591, 27.3036) -> (218.1903, 27.3036)
  line L206 (216.0966, 27.3036) -> (213.4278, 27.3036)
  line L207 (223.2403, 13.3036) -> (230.0966, 13.3036)
  line L208 (230.0966, 13.3036) -> (234.8591, 13.3036)
  line L209 (230.0966, 27.3036) -> (223.2403, 27.3036)
  line L210 (234.8591, 13.3036) -> (237.2403, 13.3036)
  line L211 (237.2403, 13.3036) -> (237.2403, 27.3036)
  line L212 (223.2403, 27.3036) -> (220.8591, 27.3036)
  line L213 (218.1903, 27.3036) -> (216.0966, 27.3036)
  line L214 (237.2403, 27.3036) -> (234.8591, 27.3036)
  line L215 (218.1903, 13.3036) -> (220.8591, 13.3036)
  line L216 (51.5028, 84.4536) -> (37.5028, 84.4536)
  line L217 (18.4528, 84.4536) -> (18.4528, 70.4536)
  line L218 (170.8528, 70.4536) -> (184.8528, 70.4536)
  line L219 (203.9028, 84.4536) -> (189.9028, 84.4536)
  line L220 (203.9028, 70.4536) -> (203.9028, 84.4536)
  line L221 (108.6528, 70.4536) -> (108.6528, 84.4536)
  line L222 (165.8028, 84.4536) -> (151.8028, 84.4536)
  line L223 (70.5528, 70.4536) -> (70.5528, 84.4536)
  line L224 (151.8028, 70.4536) -> (165.8028, 70.4536)
  line L225 (-0.5972, 84.4536) -> (-0.5972, 70.4536)
  line L226 (94.6528, 84.4536) -> (94.6528, 70.4536)
  line L227 (13.4028, 70.4536) -> (13.4028, 84.4536)
  line L228 (184.8528, 84.4536) -> (170.8528, 84.4536)
  line L229 (184.8528, 70.4536) -> (184.8528, 84.4536)
  line L230 (146.7528, 70.4536) -> (146.7528, 84.4536)
  line L231 (146.7528, 84.4536) -> (132.7528, 84.4536)
  line L232 (127.7028, 84.4536) -> (113.7028, 84.4536)
  line L233 (1.7841, 51.4036) -> (15.7841, 51.4036)
  line L234 (216.0966, 84.4536) -> (216.0966, 70.4536)
  line L235 (15.7841, 65.4036) -> (1.7841, 65.4036)
  line L236 (189.9028, 70.4536) -> (203.9028, 70.4536)
  line L237 (37.2153, 65.4036) -> (23.2153, 65.4036)
  line L238 (113.7028, 70.4536) -> (127.7028, 70.4536)
  line L239 (32.4528, 70.4536) -> (32.4528, 84.4536)
  line L240 (37.2153, 51.4036) -> (37.2153, 65.4036)
  line L241 (23.2153, 65.4036) -> (23.2153, 51.4036)
  line L242 (42.2653, 51.4036) -> (56.2653, 51.4036)
  line L243 (56.2653, 65.4036) -> (42.2653, 65.4036)
  line L244 (189.9028, 84.4536) -> (189.9028, 70.4536)
  line L245 (56.2653, 51.4036) -> (56.2653, 65.4036)
  line L246 (18.4528, 70.4536) -> (32.4528, 70.4536)
  line L247 (230.0966, 84.4536) -> (216.0966, 84.4536)
  line L248 (56.5528, 84.4536) -> (56.5528, 70.4536)
  line L249 (151.8028, 84.4536) -> (151.8028, 70.4536)
  line L250 (89.6028, 70.4536) -> (89.6028, 84.4536)
  line L251 (37.5028, 84.4536) -> (37.5028, 70.4536)
  line L252 (216.0966, 70.4536) -> (230.0966, 70.4536)
  line L253 (1.7841, 65.4036) -> (1.7841, 51.4036)
  line L254 (23.2153, 51.4036) -> (37.2153, 51.4036)
  line L255 (15.7841, 51.4036) -> (15.7841, 65.4036)
  line L256 (170.8528, 84.4536) -> (170.8528, 70.4536)
  line L257 (51.5028, 70.4536) -> (51.5028, 84.4536)
  line L258 (132.7528, 84.4536) -> (132.7528, 70.4536)
  line L259 (165.8028, 70.4536) -> (165.8028, 84.4536)
  line L260 (37.5028, 70.4536) -> (51.5028, 70.4536)
  line L261 (230.0966, 70.4536) -> (230.0966, 84.4536)
  line L262 (61.3153, 51.4036) -> (75.3153, 51.4036)
  line L263 (108.6528, 84.4536) -> (94.6528, 84.4536)
  line L264 (-0.5972, 70.4536) -> (13.4028, 70.4536)
  line L265 (70.5528, 84.4536) -> (56.5528, 84.4536)
  line L266 (113.7028, 84.4536) -> (113.7028, 70.4536)
  line L267 (56.5528, 70.4536) -> (70.5528, 70.4536)
  line L268 (65.7903, 32.3536) -> (65.7903, 46.3536)
  line L269 (141.9903, 46.3536) -> (127.9903, 46.3536)
  line L270 (156.5653, 65.4036) -> (156.5653, 51.4036)
  line L271 (127.9903, 32.3536) -> (141.9903, 32.3536)
  line L272 (141.9903, 32.3536) -> (141.9903, 46.3536)
  line L273 (75.3153, 65.4036) -> (61.3153, 65.4036)
  line L274 (170.5653, 65.4036) -> (156.5653, 65.4036)
  line L275 (118.4653, 65.4036) -> (118.4653, 51.4036)
  line L276 (122.9403, 32.3536) -> (122.9403, 46.3536)
  line L277 (42.2653, 65.4036) -> (42.2653, 51.4036)
  line L278 (75.6028, 84.4536) -> (75.6028, 70.4536)
  line L279 (89.8903, 32.3536) -> (103.8903, 32.3536)
  line L280 (75.6028, 70.4536) -> (89.6028, 70.4536)
  line L281 (89.6028, 84.4536) -> (75.6028, 84.4536)
  line L282 (127.9903, 46.3536) -> (127.9903, 32.3536)
  line L283 (13.4028, 84.4536) -> (-0.5972, 84.4536)
  line L284 (127.7028, 70.4536) -> (127.7028, 84.4536)
  line L285 (108.9403, 32.3536) -> (122.9403, 32.3536)
  line L286 (99.4153, 65.4036) -> (99.4153, 51.4036)
  line L287 (156.5653, 51.4036) -> (170.5653, 51.4036)
  line L288 (70.8403, 32.3536) -> (84.8403, 32.3536)
  line L289 (122.9403, 46.3536) -> (108.9403, 46.3536)
  line L290 (94.6528, 70.4536) -> (108.6528, 70.4536)
  line L291 (32.4528, 84.4536) -> (18.4528, 84.4536)
  line L292 (132.7528, 70.4536) -> (146.7528, 70.4536)
  line L293 (51.7903, 46.3536) -> (51.7903, 32.3536)
  line L294 (170.5653, 51.4036) -> (170.5653, 65.4036)
  line L295 (103.8903, 46.3536) -> (89.8903, 46.3536)
  line L296 (80.3653, 65.4036) -> (80.3653, 51.4036)
  line L297 (51.7903, 32.3536) -> (65.7903, 32.3536)
  line L298 (65.7903, 46.3536) -> (51.7903, 46.3536)
  line L299 (189.6153, 65.4036) -> (175.6153, 65.4036)
  line L300 (151.5153, 65.4036) -> (137.5153, 65.4036)
  line L301 (80.3653, 51.4036) -> (94.3653, 51.4036)
  line L302 (175.6153, 51.4036) -> (189.6153, 51.4036)
  line L303 (6.5466, 32.3536) -> (20.5466, 32.3536)
  line L304 (132.4653, 51.4036) -> (132.4653, 65.4036)
  line L305 (194.6653, 51.4036) -> (208.6653, 51.4036)
  line L306 (232.4778, 51.4036) -> (232.4778, 65.4036)
  line L307 (94.3653, 65.4036) -> (80.3653, 65.4036)
  line L308 (147.0403, 32.3536) -> (161.0403, 32.3536)
  line L309 (132.4653, 65.4036) -> (118.4653, 65.4036)
  line L310 (84.8403, 32.3536) -> (84.8403, 46.3536)
  line L311 (151.5153, 51.4036) -> (151.5153, 65.4036)
  line L312 (20.5466, 46.3536) -> (6.5466, 46.3536)
  line L313 (208.6653, 51.4036) -> (208.6653, 65.4036)
  line L314 (32.7403, 32.3536) -> (46.7403, 32.3536)
  line L315 (46.7403, 32.3536) -> (46.7403, 46.3536)
  line L316 (84.8403, 46.3536) -> (70.8403, 46.3536)
  line L317 (46.7403, 46.3536) -> (32.7403, 46.3536)
  line L318 (89.8903, 46.3536) -> (89.8903, 32.3536)
  line L319 (108.9403, 46.3536) -> (108.9403, 32.3536)
  line L320 (208.6653, 65.4036) -> (194.6653, 65.4036)
  line L321 (118.4653, 51.4036) -> (132.4653, 51.4036)
  line L322 (232.4778, 65.4036) -> (218.4778, 65.4036)
  line L323 (99.4153, 51.4036) -> (113.4153, 51.4036)
  line L324 (113.4153, 51.4036) -> (113.4153, 65.4036)
  line L325 (6.5466, 46.3536) -> (6.5466, 32.3536)
  line L326 (75.3153, 51.4036) -> (75.3153, 65.4036)
  line L327 (218.4778, 51.4036) -> (232.4778, 51.4036)
  line L328 (70.8403, 46.3536) -> (70.8403, 32.3536)
  line L329 (137.5153, 51.4036) -> (151.5153, 51.4036)
  point P0 (6.4028, 77.4536)